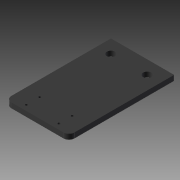
# Autodesk Inventor part: 3way_final_valve_mount
Saved by Autodesk Inventor 2019 (Build 230136000, 136)
## iProperties
Created: 2019-08-14
Part Number: 3way_final_valve_mount
Material: Generic
Document SubType Name: Modeling
Designer: devon
Density: 1 g/cm^3
Appearance: Default
Author: devon
Autodesk Inventor part; units mm, degrees
ref_plane "YZ Plane" through (0, 0, 0) normal (1, 0, 0) x (0, 1, 0)
ref_plane "XZ Plane" through (0, 0, 0) normal (0, 1, 0) x (-1, 0, 0)
ref_plane "XY Plane" through (0, 0, 0) normal (0, 0, 1) x (1, 0, 0)
sketch "Sketch1" plane through (0, 0, 0) normal (0, 1, 0) x (-1, 0, 0)
  line L0 (30, 50) -> (-30, 50)
  line L1 (-30, 50) -> (-30, -50)
  line L2 (-30, -50) -> (30, -50)
  line L3 (30, -50) -> (30, 50)
  line L4 (30, 50) -> (-30, -50) construction
  line L5 (-30, 50) -> (30, -50) construction
  point P0 (0, 0)
  dimension "d0" = 60
  dimension "d1" = 100
  constraints: 12 end point, 2 midpoint, 2 parallel, 1 horizontal, 1 perpendicular
  measures "d0" distance of L1.end L2.end
  measures "d1" distance of L2.end L0.start
extrude "Extrusion1" add sketch "Sketch1" along normal blind 5
sketch "Sketch2" plane through (0, 5, 0) normal (0, 1, 0) x (1, 0, 0)
  circle A0 centre (15.5, -45) radius 1.25
  circle A1 centre (15.5, -32.3) radius 1.25
  line L0 (-30, -50) -> (30, -50) projected
  line L1 (30, -50) -> (30, 50) projected
  circle A2 centre (-15.5, -45) radius 1.25
  line L2 (-30, 50) -> (-30, -50) projected
  circle A3 centre (-15.5, -32.3) radius 1.25
  point P0 (0, 0)
  dimension "d4" = 2.5
  dimension "d5" = 2.5
  dimension "d6" = 12.7
  dimension "d7" = 5
  dimension "d8" = 14.5
  dimension "d9" = 14.5
  dimension "d10" = 2.5
  dimension "d11" = 14.5
  dimension "d12" = 2.5
  constraints: 4 centre point
  measures "d4" diameter of A1
  measures "d5" diameter of A0
  measures "d6" distance of A1.centre A0.centre
  measures "d7" distance from line of L0 A0.centre
  measures "d8" distance from line of L1 A0.centre
  measures "d9" distance from line of L1 A1.centre
  measures "d10" diameter of A2
  measures "d11" distance from line of L2 A2.centre
  measures "d12" diameter of A3
extrude "Extrusion2" cut sketch "Sketch2" against normal up to next
sketch "Sketch3" plane through (0, 5, 0) normal (0, 1, 0) x (1, 0, 0)
  circle A0 centre (-17.3, 37.3) radius 4
  line L0 (30, 50) -> (-30, 50) projected
  line L1 (-30, 50) -> (-30, -50) projected
  circle A1 centre (17.3, 37.3) radius 4
  line L2 (30, -50) -> (30, 50) projected
  point P0 (0, 0)
  dimension "d15" = 8
  dimension "d16" = 12.7
  dimension "d17" = 12.7
  dimension "d18" = 8
  dimension "d19" = 12.7
  constraints: 2 centre point
  measures "d15" diameter of A0
  measures "d16" distance from line of L0 A0.centre
  measures "d17" distance from line of L1 A0.centre
  measures "d18" diameter of A1
  measures "d19" distance from line of L2 A1.centre
extrude "Extrusion3" cut sketch "Sketch3" against normal up to next
fillet "Fillet1" radius 5 2 edges at (30, 2.5, 50) (-30, 2.5, 50)
body "Solid1"
